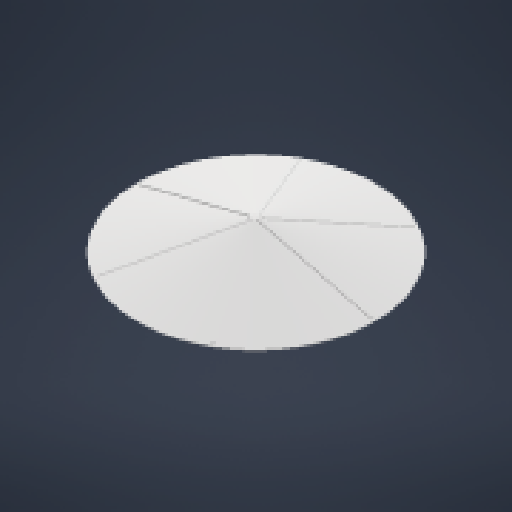
# Autodesk Inventor part: central disk
Saved by Autodesk Inventor 2026 (Build 300175050, 175E)
## iProperties
Created: 2026-03-26
Part Number: central disk
Material: Generic
Document SubType Name: Modeling
Designer: sniel
Density: 1 g/cm^3
Appearance: Default
Author: sniel
Autodesk Inventor part; units mm, degrees
ref_plane "YZ Plane" through (0, 0, 0) normal (1, 0, 0) x (0, 1, 0)
ref_plane "XZ Plane" through (0, 0, 0) normal (0, 1, 0) x (-1, 0, 0)
ref_plane "XY Plane" through (0, 0, 0) normal (0, 0, 1) x (1, 0, 0)
sketch "Sketch1" plane through (0, 0, 0) normal (0, 0, 1) x (1, 0, 0)
  line L0 (-80, 33) -> (0, 53)
  line L1 (-80, 33) -> (-80, 28)
  line L2 (0, 53) -> (0, 48)
  line L3 (0, 48) -> (-80, 28)
  line L4 (0, 53) -> (0, 48)
  line L5 (0, -10.6) -> (0, 63.6) projected
  line L6 (0, 53) -> (-2.5, 53)
  line L7 (-2.5, 53) -> (-2.5, 28)
  line L8 (-2.5, 28) -> (0, 28)
  line L9 (0, 28) -> (0, 53)
  line L10 (-80, 30.5) -> (0, 50.5)
  line L11 (-2.5, 28) -> (0, 28)
  line L12 (0, 28) -> (0, 8)
  line L13 (0, 8) -> (-2.5, 8)
  line L14 (-2.5, 8) -> (-2.5, 28)
  line L15 (-80, 30.5) -> (-78, 28.5)
  line L16 (-80, 30.5) -> (-77.1716, 30.5) construction
  line L17 (-80, 33) -> (-78, 31)
  line L18 (-80, 33) -> (-77.1716, 33) construction
  point P0 (0, 0)
  point P1 (-2.5, 47.375)
  point P2 (-2.5, 49.875)
  dimension "d2" = 5
  dimension "d3" = 5
  dimension "d5" = 2.5
  dimension "d11" = 20
  dimension "d24" = 45
  dimension "d25" = 45
  constraints: 36 end point, 4 horizontal, 4 parallel, 4 point on line, 2 equal length, 2 perpendicular, 2 vertical, 1 midpoint
  measures "d2" distance of L0.start L1.end
  measures "d3" distance of L0.end L2.end
  measures "d5" distance of L8.end L7.end
  measures "d11" distance of L11.end L12.end
  measures "d24" angle of L15 L16
  measures "d25" angle of L17 L18
revolve "Revolution1" add sketch "Sketch1" angle 360 about axis through (0, -10, 0) along (0, 1, 0) contours L0 L7 L10 L17 | L0 L2 L10 L7 | L10 L2 L3 L7 | L3 L5 L8 L7 | L8 L5 L13 L14
sketch "Sketch3" plane through (0, 0, 0) normal (0, 0, 1) x (1, 0, 0)
  line L0 (-1, 3) -> (1, 3)
  line L1 (1, 3) -> (1, 13)
  line L2 (1, 13) -> (-1, 13)
  line L3 (-1, 13) -> (-1, 3)
  line L4 (2.5, 8) -> (-2.5, 8) projected
  line L5 (-1, 3) -> (1, 13) construction
  line L6 (1, 3) -> (-1, 13) construction
  point P0 (0, 0)
  point P1 (0, 8)
  constraints: 12 end point, 3 midpoint, 2 parallel, 1 horizontal, 1 perpendicular
extrude "Extrusion2" cut sketch "Sketch3" along normal mid plane 16.75
sketch "Sketch4" plane through (0, 0, 0) normal (0, 0, 1) x (1, 0, 0)
  line L0 (-80, 33) -> (0, 53) projected
  line L1 (0, 53) -> (-80, 33)
  line L2 (0, 53) -> (0, 55)
  line L3 (0, 55) -> (-80, 35)
  line L4 (-80, 35) -> (-80, 33)
  line L5 (-80, 33) -> (-78.0597, 33.4851)
  line L6 (-78.0597, 33.4851) -> (-78.0597, 35.4851)
  line L7 (-80, 34) -> (0, 54)
  point P0 (0, 0)
  point P1 (-78.0597, 34.4851)
  dimension "d14" = 2
  dimension "d15" = 2
  constraints: 14 end point, 4 point on line, 2 midpoint, 2 parallel, 2 vertical
  measures "d14" distance of L1.start L2.end
  measures "d15" distance of L1.end L5.end
extrude "Extrusion3" add sketch "Sketch4" along normal mid plane 2 contours L6 L7 L2 L0
pattern_circular "Circular Pattern2" count 6 over 360 about axis through (0, -10, 0) along (0, 1, 0) of "Extrusion3"
sketch "Sketch5" plane through (0, 0, 0) normal (0, 0, 1) x (1, 0, 0)
  line L0 (-3.2364, 54.433) -> (3.2364, 54.433)
  line L1 (3.2364, 54.433) -> (3.2364, 53.567)
  line L2 (3.2364, 53.567) -> (-3.2364, 53.567)
  line L3 (-3.2364, 53.567) -> (-3.2364, 54.433)
  line L4 (0, 54) -> (0.5774, 53.8557) projected
  line L5 (-3.2364, 54.433) -> (3.2364, 53.567) construction
  line L6 (3.2364, 54.433) -> (-3.2364, 53.567) construction
  point P0 (0, 0)
  constraints: 12 end point, 2 midpoint, 2 parallel, 1 horizontal, 1 perpendicular
extrude "Extrusion4" cut sketch "Sketch5" along normal mid plane 4.75
sketch "Sketch6" plane through (0, 0, 0) normal (0, 0, 1) x (1, 0, 0)
  line L0 (-78, 31) -> (-80, 33) projected
  line L1 (-80, 33) -> (0, 33)
  line L2 (78, 31) -> (-78, 31) projected
  line L3 (0, 33) -> (0, 31)
  line L4 (-78, 31) -> (0, 31)
  point P0 (0, 0)
  constraints: 6 end point, 1 midpoint, 1 parallel, 1 perpendicular
extrude "Extrusion5" add sketch "Sketch6" along normal mid plane 4.75
pattern_circular "Circular Pattern3" count 6 over 360 about axis through (0, -10, 0) along (0, 1, 0) of "Extrusion5"
body "Solid1"
